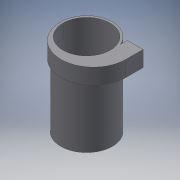
# Autodesk Inventor part: Main Cyclone
Saved by Autodesk Inventor 2018 (Build 220112000, 112)
## iProperties
Created: 2018-02-05
Part Number: Main Cyclone
Material: Generic
Document SubType Name: Modeling
Designer: Rus
Density: 1 g/cm^3
Appearance: Default
Author: Rus
Autodesk Inventor part; units mm, degrees
ref_plane "YZ Plane" through (0, 0, 0) normal (1, 0, 0) x (0, 1, 0)
ref_plane "XZ Plane" through (0, 0, 0) normal (0, 1, 0) x (-1, 0, 0)
ref_plane "XY Plane" through (0, 0, 0) normal (0, 0, 1) x (1, 0, 0)
sketch "Sketch1" plane through (0, 0, 0) normal (0, 1, 0) x (-1, 0, 0)
  circle A0 centre (0, 0) radius 76.2
  circle A1 centre (0, 0) radius 69.85
  dimension "d1" = 152.4
  dimension "d6" = 6.35
  constraints: 2 centre point, 2 coincident
  measures "d1" diameter of A0
  measures "d6" radial gap between concentric circles of A0 A1
extrude "Extrusion1" add sketch "Sketch1" against normal blind 152.4
sketch "Sketch18" plane through (0, 0, 0) normal (0, 1, 0) x (1, 0, 0)
  circle A0 centre (0, 0) radius 69.85 construction
  circle A1 centre (0, 0) radius 76.2 construction
  line L0 (110.0667, 0) -> (110.0667, 50.8)
  line L1 (110.0667, 50.8) -> (116.4167, 50.8)
  line L2 (116.4167, 50.8) -> (116.4167, 0)
  arc A2 (-76.2, 0) -> (116.4167, 0) centre (20.1083, 0) ccw
  arc A3 (-69.85, 0) -> (110.0667, 0) centre (20.1083, 0) ccw
  circle A4 centre (0, 0) radius 76.2 construction
  circle A5 centre (0, 0) radius 69.85 construction
  arc A6 (69.85, 30.4535) -> (-76.2, 0) centre (0, 0) ccw
  arc A7 (69.85, 0) -> (-69.85, 0) centre (0, 0) ccw
  line L3 (76.2, 0) -> (76.2, 50.8)
  line L4 (76.2, 50.8) -> (69.85, 50.8)
  line L5 (69.85, 50.8) -> (69.85, 30.4535)
  line L6 (69.85, 0) -> (0, 0) construction
  line L7 (76.2, 0) -> (69.85, 0)
  dimension "d79" = 6.35
  dimension "d80" = 50.8
  dimension "d86" = 33.8667
  dimension "d88" = 6.35
  constraints: 16 end point, 13 point on circle, 5 horizontal alignment, 5 tangent, 4 centre point, 3 perpendicular, 3 vertical, 2 coincident, 2 equal length, 1 concentric, 1 horizontal, 2 other
  measures "d79" distance of L0.end L1.end
  measures "d80" distance of L1.end L2.end
  measures "d86" distance of L3.end L0.end
  measures "d88" distance of L3.start L7.end
extrude "Extrusion14" add sketch "Sketch18" along normal blind 33.8667
sketch "Sketch19" plane through (0, 0, 0) normal (0, -1, 0) x (1, 0, 0)
  arc A0 (-46.7895, 60.143) -> (-76.2, 0) centre (0, 0) ccw projected
  arc A1 (110.0667, 0) -> (-46.7895, 60.143) centre (20.1083, 0) ccw projected
  line L0 (110.0667, 0) -> (110.0667, -50.8) projected
  line L1 (110.0667, -50.8) -> (116.4167, -50.8) projected
  line L2 (116.4167, -50.8) -> (116.4167, 0) projected
  arc A2 (116.4167, 0) -> (-76.2, 0) centre (20.1083, 0) ccw projected
  line L3 (69.85, -50.8) -> (69.85, -30.4535) projected
  arc A3 (69.85, -30.4535) -> (76.2, 0) centre (0, 0) ccw projected
  line L4 (69.85, -30.4535) -> (69.85, -50.8) projected
  line L5 (69.85, -50.8) -> (76.2, -50.8) projected
  line L6 (76.2, -50.8) -> (76.2, 0) projected
  line L7 (110.0667, -50.8) -> (76.2, -50.8)
  arc A4 (76.2, 0) -> (-46.7895, 60.143) centre (0, 0) ccw projected
  constraints: 2 end point, 1 horizontal
extrude "Extrusion15" add sketch "Sketch19" along normal blind 6.35
sketch "Sketch21" plane through (0, 33.8667, 0) normal (0, 1, 0) x (1, 0, 0)
  arc A0 (-69.85, 0) -> (110.0667, 0) centre (20.1083, 0) ccw projected
  arc A1 (69.85, 0) -> (-69.85, 0) centre (0, 0) ccw projected
  line L0 (69.85, 0) -> (76.2, 0) projected
  line L1 (76.2, 0) -> (76.2, 50.8) projected
  line L2 (76.2, 50.8) -> (69.85, 50.8) projected
  line L3 (69.85, 50.8) -> (69.85, 30.4535) projected
  arc A2 (69.85, 30.4535) -> (-76.2, 0) centre (0, 0) ccw projected
  arc A3 (-76.2, 0) -> (116.4167, 0) centre (20.1083, 0) ccw projected
  line L4 (116.4167, 0) -> (116.4167, 50.8) projected
  line L5 (116.4167, 50.8) -> (110.0667, 50.8) projected
  line L6 (110.0667, 50.8) -> (110.0667, 0) projected
  arc A4 (-69.85, 0) -> (69.85, 0) centre (0, 0) ccw
  line L7 (110.0667, 50.8) -> (76.2, 50.8)
  constraints: 2 end point, 2 point on circle, 1 centre point, 1 coincident, 1 horizontal
extrude "Extrusion17" add sketch "Sketch21" along normal blind 6.35 contours A4 L0 L1 L7 L6 A0 | A0 L6 L5 L4 A3 A2 L3 L2 L1 L0 A1
chamfer "Chamfer1" distance 6.35 distance2 12.7 1 edges at (76.2, 16.9333, 0) measured on face at (74.0833, 11.2889, 0)
fillet "Fillet1" radius 36.5125 1 edges at (76.2, 16.9333, -12.6995)
body "Solid1"
